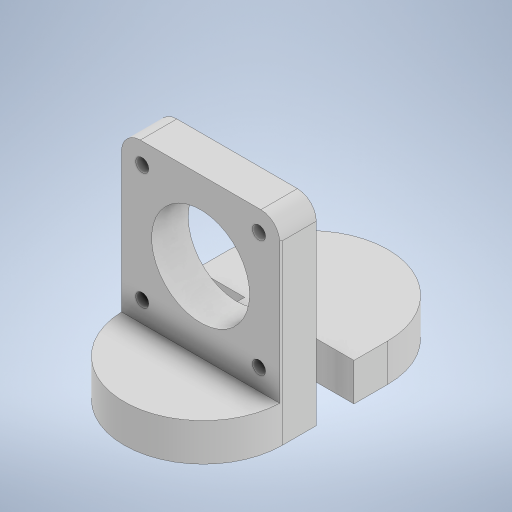
# Autodesk Inventor part: tete_v2
Saved by Autodesk Inventor 2024.1 (Build 281209000, 209)
## iProperties
Created: 2024-04-06
Part Number: tete_v2
Material: Générique
Document SubType Name: Modeling
Designer: chass
Density: 1 g/cm^3
Appearance: Par défaut
Author: chass
Autodesk Inventor part; units mm, degrees
ref_plane "YZ Plane" through (0, 0, 0) normal (1, 0, 0) x (0, 1, 0)
ref_plane "XZ Plane" through (0, 0, 0) normal (0, 1, 0) x (-1, 0, 0)
ref_plane "XY Plane" through (0, 0, 0) normal (0, 0, 1) x (1, 0, 0)
sketch "Esquisse1" plane through (0, 0, 0) normal (0, 1, 0) x (-1, 0, 0)
  circle A0 centre (0, 25) radius 4.2
  line L0 (16, 0) -> (-13, 0)
  circle A1 centre (0, -25) radius 4.2
  line L1 (21, 5) -> (-21, 5)
  line L2 (-21, 5) -> (-21, -5)
  line L3 (-21, -5) -> (21, -5)
  line L4 (21, -5) -> (21, 5)
  line L5 (21, 5) -> (-21, -5)
  line L6 (-21, 5) -> (21, -5)
  line L7 (8, 5) -> (-8, 5)
  line L8 (-8, 5) -> (-8, -5)
  line L9 (-8, -5) -> (8, -5)
  line L10 (8, -5) -> (8, 5)
  line L11 (8, 5) -> (-8, -5)
  line L12 (-8, 5) -> (8, -5)
  line L13 (21, 5) -> (21, 35)
  line L14 (-21, 35) -> (-21, 5)
  line L15 (21, 35) -> (-21, 35)
  line L16 (21, -5) -> (21, -35)
  line L17 (-21, -35) -> (-21, -5)
  line L18 (21, -35) -> (-21, -35)
  point P0 (0, 0)
  point P1 (0, 0)
  point P2 (0, 0)
  point P3 (8, -5)
  point P4 (-8, 5)
  dimension "d0" = 8.4
  dimension "d1" = 25
  dimension "d2" = 42
  dimension "d3" = 10
  dimension "d4" = 16
  constraints: 38 end point, 4 horizontal, 4 parallel, 3 midpoint, 3 symmetric about line, 2 centre point, 2 perpendicular, 1 coincident, 1 point on line, 1 vertical, 1 other
  measures "d0" diameter of A0
  measures "d1" distance of point (0, 0) A0.centre
  measures "d2" distance of L2.end L3.end
  measures "d3" distance of L3.end L1.start
  measures "d4" distance between parallel lines of L8 L10
extrude "Extrusion1" add sketch "Esquisse1" along normal blind 10 contours L10 L6 L0 | L0 L5 L10 | L5 L8 L0 | L11 L10 L5 | L11 L8 L5 | L0 L8 L6 | L12 L1 L11 | L12 L3 L11 | L6 L8 L12 | L6 L10 L12 | L1 L14 L15 L13 | L3 L16 L18 L17
sketch "Esquisse2" plane through (0, 10, 0) normal (0, 1, 0) x (1, 0, 0)
  line L0 (-8, -5) -> (-21, -5) projected
  line L1 (-21, -5) -> (21, -5)
  line L2 (21, -5) -> (21, -14.7)
  line L3 (21, -14.7) -> (-21, -14.7)
  line L4 (-21, -14.7) -> (-21, -5)
  point P0 (0, 0)
  dimension "d8" = 9.7
  dimension "d9" = 42
  constraints: 8 end point, 2 parallel, 1 horizontal, 1 perpendicular
  measures "d8" distance of L3.end L0.end
  measures "d9" distance of L2.end L3.end
extrude "Extrusion2" add sketch "Esquisse2" along normal blind 42
sketch "Esquisse3" plane through (0, 10, 0) normal (0, 1, 0) x (1, 0, 0)
  line L0 (21, -14.7) -> (-21, -14.7) projected
  line L1 (-21, -35) -> (21, -35)
  line L2 (21, -35) -> (21, -14.7)
  line L3 (21, -14.7) -> (-21, -14.7)
  line L4 (-21, -14.7) -> (-21, -35)
  line L5 (21, 35) -> (-21, 35) projected
  line L6 (-21, 5) -> (21, 5)
  line L7 (21, 5) -> (21, 35)
  line L8 (21, 35) -> (-21, 35)
  line L9 (-21, 35) -> (-21, 5)
  point P0 (0, 0)
  point P1 (-21, -14.7)
  constraints: 16 end point, 4 parallel, 2 horizontal, 2 perpendicular, 1 point on line
extrude "Extrusion3" add sketch "Esquisse3" against normal blind 2
sketch "Esquisse4" plane through (-21, 10, 14.7) normal (0, 0, 1) x (1, 0, 0)
  line L0 (42, 42) -> (0, 42) projected
  line L1 (42, 0) -> (0, 0)
  line L2 (0, 0) -> (42, 42)
  circle A0 centre (21, 21) radius 13
  line L3 (5.5, 5.5) -> (36.5, 5.5)
  line L4 (36.5, 5.5) -> (36.5, 36.5)
  line L5 (36.5, 36.5) -> (5.5, 36.5)
  line L6 (5.5, 36.5) -> (5.5, 5.5)
  line L7 (5.5, 36.5) -> (36.5, 5.5)
  circle A1 centre (5.5, 36.5) radius 1.75
  circle A2 centre (5.5, 5.5) radius 1.75
  line L8 (21, 36.5) -> (21, 5.5)
  circle A3 centre (36.5, 36.5) radius 1.75
  circle A4 centre (36.5, 5.5) radius 1.75
  point P0 (21, -10)
  point P1 (36.5, 5.5)
  dimension "d14" = 26
  dimension "d20" = 31
  dimension "d21" = 3.5
  dimension "d22" = 3.5
  constraints: 16 end point, 5 centre point, 4 midpoint, 3 parallel, 3 point on line, 3 symmetric about line, 1 coincident, 1 horizontal, 1 perpendicular, 2 other
  measures "d14" diameter of A0
  measures "d20" distance of L4.end L5.end
  measures "d21" diameter of A1
  measures "d22" diameter of A2
extrude "Extrusion4" cut sketch "Esquisse4" against normal blind 10 contours A2 L6 L2 | L2 L3 A2 | L6 A2 L2 | L2 A2 L3 | A1 L5 L6 | L6 L7 A1 | A0 L7 L2 | L2 L8 A0 | L5 A1 L7 | A4 L7 L3 | L3 L4 A4 | L8 L7 A0 | L8 A0 L2 | L2 A0 L7 | L7 A0 L8 | L7 A4 L4 | A3 L2 L5 | L5 L2 A3 | L2 L4 A3 | L2 A3 L4
fillet "Congé1" radius 5 2 edges at (21, 52, 9.85) (-21, 52, 9.85)
fillet "Congé2" radius 21 4 edges at (21, 5, -35) (-21, 5, -35) (21, 5, 35) (-21, 5, 35)
